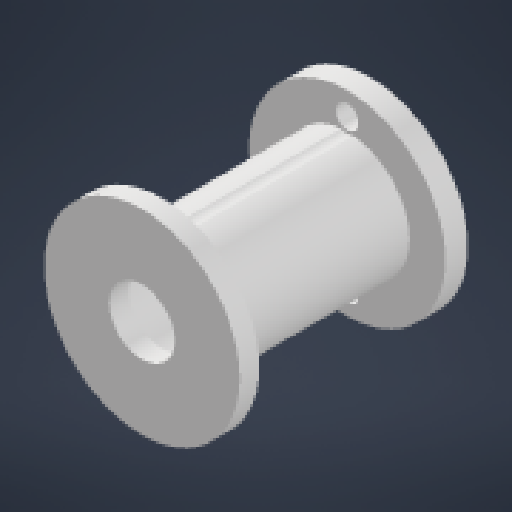
# Autodesk Inventor part: TeceraParte
Saved by Autodesk Inventor 2026.3 (Build 303398000, 398)
## iProperties
Created: 2026-07-23
Part Number: TeceraParte
Material: Genérico
Document SubType Name: Modeling
Designer: ASUS
Density: 1 g/cm^3
Appearance: Valor por defecto
Author: ASUS
Autodesk Inventor part; units mm, degrees
ref_plane "YZ Plane" through (0, 0, 0) normal (1, 0, 0) x (0, 1, 0)
ref_plane "XZ Plane" through (0, 0, 0) normal (0, 1, 0) x (-1, 0, 0)
sketch "Boceto1" plane through (0, 0, 0) normal (0, 0, 1) x (1, 0, 0)
  circle A0 centre (-8.5, 0) radius 8.65
  circle A1 centre (-8.5, -11.5) radius 1.75
  circle A2 centre (-8.5, 11.5) radius 1.75
  circle A3 centre (-8.5, 0) radius 14.5
  circle A4 centre (-8.5, 0) radius 14.5
  circle A5 centre (-8.5, 0) radius 9.5
  circle A6 centre (-8.5, -11.5) radius 2.25
  circle A7 centre (-8.5, 11.5) radius 2.25
  point P0 (0, 0)
  dimension "d0" = 17.3
  dimension "d1" = 3.5
  dimension "d2" = 3.5
  dimension "d3" = 19
  dimension "d4" = 4.5
  dimension "d5" = 4.5
  constraints: 8 centre point, 7 coincident, 1 concentric
  measures "d0" diameter of A0
  measures "d1" diameter of A1
  measures "d2" diameter of A2
  measures "d3" diameter of A5
  measures "d4" diameter of A6
  measures "d5" diameter of A7
sketch "Boceto2" plane through (0, 0, 0) normal (0, 0, 1) x (1, 0, 0)
  arc A0 (6.4812, 0.75) -> (6.4812, -0.75) centre (-8.5, 0) ccw projected
  circle A1 centre (-8.5, 0) radius 15
  point P0 (0, 0)
  point P1 (6.4812, -0.75)
  point P2 (6.4812, 0.75)
  constraints: 1 centre point, 1 coincident, 1 concentric
extrude "Extrusión1" add sketch "Boceto2" along normal blind 3.5
sketch "Boceto3" plane through (-8.5, 0, 3.5) normal (0, 0, 1) x (1, 0, 0)
  circle A0 centre (0, -11.5) radius 1.75 projected
  circle A1 centre (0, -11.5) radius 2.25 projected
  circle A2 centre (0, 0) radius 9.5 projected
  circle A3 centre (0, 0) radius 8.65 projected
  circle A4 centre (0, 11.5) radius 2.25 projected
  circle A5 centre (0, 11.5) radius 1.75 projected
  point P0 (8.5, 0)
  point P1 (0.9357, 9.4538)
  point P2 (-0.9357, 9.4538)
  point P3 (-0.9357, -9.4538)
  point P4 (0.9357, -9.4538)
sketch "Boceto4" plane through (-8.5, 0, 3.5) normal (0, 0, 1) x (1, 0, 0)
  circle A0 centre (0, 0) radius 5
  point P0 (8.5, 0)
  dimension "d8" = 10
  constraints: 1 centre point
  measures "d8" diameter of A0
extrude "Extrusión2" cut sketch "Boceto4" against normal blind 10
ref_plane "Plano de trabajo1" through (-16.5, -8, 30) normal (0, 0, 1) x (1, 0, 0)
extrude "Extrusión3" add sketch "Boceto3" along normal up to surface (26.5 mm away) contours A1 A2 A4
extrude "Extrusión4" cut sketch "Boceto1" along normal blind 10 contours A1 | A2
sketch "Boceto5" plane through (-8.5, 11.5, 30) normal (0, 0, 1) x (1, 0, 0)
  arc A0 (0.9357, -20.9538) -> (0.9357, -2.0462) centre (0, -11.5) ccw projected
  arc A1 (-0.9357, -2.0462) -> (-0.9357, -20.9538) centre (0, -11.5) ccw projected
  arc A2 (-0.9357, -2.0462) -> (0.9357, -2.0462) centre (0, 0) ccw projected
  arc A3 (0.9357, -20.9538) -> (-0.9357, -20.9538) centre (0, -23) ccw projected
  circle A4 centre (0, -11.5) radius 8.65 projected
  point P0 (8.5, -11.5)
extrude "Extrusión5" add sketch "Boceto5" along normal blind 2
sketch "Boceto6" plane through (-8.5, 11.5, 32) normal (0, 0, 1) x (1, 0, 0)
  circle A0 centre (0, -11.5) radius 15 projected
  circle A1 centre (0, -11.5) radius 5 projected
  circle A2 centre (0, -11.5) radius 5 projected
  point P0 (8.5, -11.5)
extrude "Extrusión6" add sketch "Boceto6" along normal blind 3
sketch "Boceto7" plane through (-8.5, 0, 0) normal (0, 0, -1) x (-1, 0, 0)
  circle A0 centre (0, 0) radius 5 projected
  circle A1 centre (0, 0) radius 8.65
  point P0 (-8.5, 0)
  dimension "d19" = 17.3
  constraints: 1 centre point, 1 coincident
  measures "d19" diameter of A1
extrude "Extrusión7" cut sketch "Boceto7" against normal blind 10 contours A0 | A1
